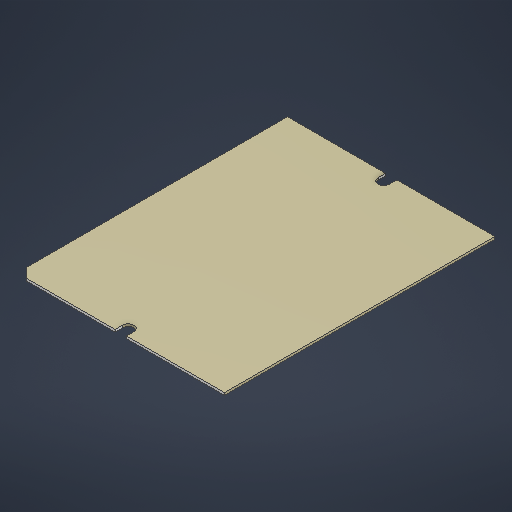
# Autodesk Inventor part: etl standard baseplate with cutouts
Saved by Autodesk Inventor 2027 (Build 310192060, 192F)
## iProperties
Created: 2021-07-27
Part Number: etl standard baseplate with cutouts
Material: Generic
Document SubType Name: Modeling
Designer: Caleb
Density: 1 g/cm^3
Appearance: Default
Sending System: Autodesk Inventor 2022
Preprocessor: ST-DEVELOPER v18.1
Title: C:\Users\Caleb\Desktop\etl standard baseplate.stp
Author: Caleb
Autodesk Inventor part; units mm, degrees
ref_plane "YZ Plane" through (0, 0, 0) normal (1, 0, 0) x (0, 1, 0)
ref_plane "XZ Plane" through (0, 0, 0) normal (0, 1, 0) x (-1, 0, 0)
ref_plane "XY Plane" through (0, 0, 0) normal (0, 0, 1) x (1, 0, 0)
sketch "Sketch2" plane through (0, 0, 0) normal (0, 1, 0) x (-1, 0, 0)
  line L0 (-22.05, -28.75) -> (22.05, -28.75)
  line L1 (22.05, -28.75) -> (22.05, 28.75)
  line L2 (22.05, 28.75) -> (-22.05, 28.75)
  line L3 (-22.05, 28.75) -> (-22.05, -28.75)
  line L4 (-22.05, -28.75) -> (22.05, 28.75) construction
  line L5 (22.05, -28.75) -> (-22.05, 28.75) construction
  point P0 (0, 0)
  dimension "d28" = 44.1
  dimension "d29" = 57.5
  constraints: 12 end point, 2 midpoint, 2 parallel, 1 horizontal, 1 perpendicular
  measures "d28" distance of L1.end L2.end
  measures "d29" distance of L0.end L1.end
extrude "Extrusion2" add sketch "Sketch2" along normal blind 0.5
sketch "Sketch4" plane through (0, 0.5, 0) normal (0, 1, 0) x (1, 0, 0)
  line L0 (-22.05, 28.75) -> (-22.05, -28.75) projected
  line L1 (-22.05, -28.75) -> (22.05, -28.75) projected
  line L2 (22.05, -28.75) -> (22.05, 28.75) projected
  line L3 (22.05, 28.75) -> (-22.05, 28.75) projected
  point P0 (0, 0)
  point P1 (0, -27.15)
  point P2 (0, 27.15)
  point P3 (-18, -28.75)
  point P4 (-12.775, 28.75)
  dimension "d37" = 22.05
  dimension "d38" = 1.6
  dimension "d40" = 1.6
  dimension "d68" = 44.1
  constraints: 1 vertical alignment
  measures "d37" distance from line of L0 point (0, -27.15)
  measures "d38" distance from line of L1 point (0, -27.15)
  measures "d40" distance from line of L3 point (0, 27.15)
  measures "d68" distance of L0.end L1.end
hole "Hole1" at (0, 0.5, 27.15) at (0, 0.5, -27.15) direction (0, -1, 0) diameter 2.4 end through all clearance for "Flat Head Machine Screw" size "M2" standard "Ansi Metric M Profile"
sketch "Sketch5" plane through (0, 0.5, 0) normal (0, 1, 0) x (1, 0, 0)
  line L0 (-22.05, -28.75) -> (22.05, -28.75) projected
  line L1 (-20.05, -28.75) -> (-22.05, -26.75)
  line L2 (-22.05, 28.75) -> (-22.05, -28.75) projected
  point P0 (0, 0)
  point P1 (-18, -28.75)
  dimension "d49" = 2
  dimension "d50" = 2
  constraints: 2 end point, 2 point on line
  measures "d49" distance of L0.start L1.start
  measures "d50" distance of L0.start L1.end
extrude "Extrusion4" cut sketch "Sketch5" against normal through all
sketch "Sketch6" plane through (0, 0.5, 0) normal (0, 1, 0) x (1, 0, 0)
  circle A0 centre (0, -27.15) radius 1.2 projected
  line L0 (-1.2, -27.15) -> (-1.2, -28.75)
  line L1 (-22.05, -28.75) -> (22.05, -28.75) projected
  line L2 (1.2, -27.15) -> (1.2, -28.75)
  line L3 (1.2, -27.15) -> (-1.2, -27.15)
  line L4 (24.0299, 0) -> (-42.1887, 0)
  line L5 (-1.2, 27.15) -> (-1.2, 28.75)
  line L6 (1.2, 27.15) -> (1.2, 28.75)
  line L7 (1.2, 27.15) -> (-1.2, 27.15)
  line L8 (22.05, 28.75) -> (-22.05, 28.75) projected
  point P0 (0, 0)
  point P1 (-15.5, -28.75)
  point P2 (17.3, -28.75)
  point P3 (0, 27.15)
  point P4 (15.5, 28.75)
  point P5 (-17.3, 28.75)
  constraints: 14 end point, 5 symmetric about line, 2 horizontal, 2 horizontal alignment, 2 point on circle, 2 point on line, 2 vertical
extrude "Extrusion5" cut sketch "Sketch6" against normal through all contours L2 L1 L0 A0 | L5 L8 L6 L7
equation "\"d37\" = 0.5 * d68"
equation "\"d40\" = d38"
body "Solid3"
